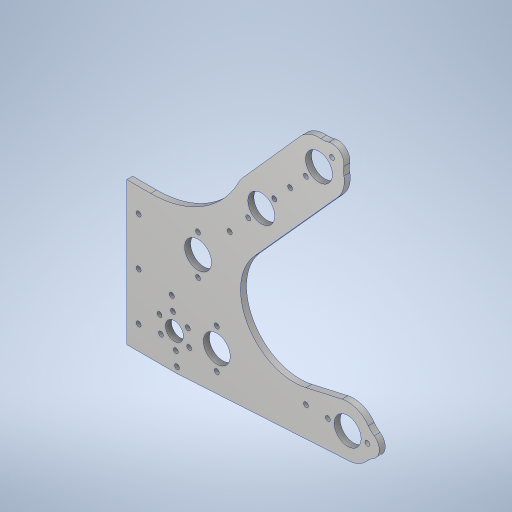
# Autodesk Inventor part: GP8-002
Saved by Autodesk Inventor 2023.4 (Build 274418000, 418)
## iProperties
Created: 2025-02-26
Part Number: GP8-002
Material: Aluminum 6061
Document SubType Name: Modeling
Designer: dlangdon
Density: 2.7 g/cm^3
Appearance: Aluminum - Flat
Author: dlangdon
Autodesk Inventor part; units mm, degrees
ref_plane "YZ Plane" through (0, 0, 0) normal (1, 0, 0) x (0, 1, 0)
ref_plane "XZ Plane" through (0, 0, 0) normal (0, 1, 0) x (-1, 0, 0)
ref_plane "XY Plane" through (0, 0, 0) normal (0, 0, 1) x (1, 0, 0)
sketch "Sketch1" plane through (0, 0, 0) normal (0, 0, 1) x (1, 0, 0)
  line L0 (0, 0) -> (704.681, 0) construction
  line L1 (704.681, 0) -> (704.681, 101.6) construction
  line L2 (704.681, 101.6) -> (0, 101.6) construction
  circle A0 centre (304.8, 38.1) radius 38.1 construction
  circle A1 centre (212.725, 197.5786) radius 38.1 construction
  circle A2 centre (274.2046, 266.7) radius 38.1 construction
  circle A3 centre (499.5893, 180.5177) radius 203.2 construction
  line L3 (78.3329, 304.8) -> (550.894, 304.8) construction
  circle A4 centre (247.764, 111.4893) radius 57.15 construction
  circle A5 centre (258.7625, 117.8393) radius 53.975 construction
  line L4 (212.725, 197.5786) -> (304.8, 38.1) construction
  line L5 (258.7625, 117.8393) -> (247.764, 111.4893) construction
  line L6 (274.2046, 266.7) -> (212.725, 197.5786) construction
  dimension "d0" = 101.6
  dimension "d2" = 76.2
  dimension "d3" = 76.2
  dimension "d4" = 76.2
  dimension "d8" = 406.4
  dimension "d9" = 304.8
  dimension "d11" = 304.8
  dimension "d13" = 114.3
  dimension "d14" = 107.95
  dimension "d15" = 12.7
  dimension "d16" = 92.5068
  dimension "d17" = 60
  constraints: 14 end point, 6 centre point, 6 tangent, 3 perpendicular, 2 horizontal, 1 midpoint
  measures "d0" distance of L0.end L1.end
  measures "d2" diameter of A0
  measures "d3" diameter of A1
  measures "d4" diameter of A2
  measures "d8" diameter of A3
  measures "d9" distance between parallel lines of L0 L3
  measures "d11" horizontal distance of L4.end L0.start
  measures "d13" diameter of A4
  measures "d14" diameter of A5
  measures "d15" distance of L5.start L5.end
  measures "d16" distance of L6.start L4.start
  measures "d17" angle of L0 L4
sketch "Sketch4" plane through (0, 0, 0) normal (0, 0, 1) x (1, 0, 0)
  circle A0 centre (274.2046, 266.7) radius 38.1 construction
  circle A1 centre (212.725, 197.5786) radius 38.1 construction
  circle A2 centre (247.764, 111.4893) radius 57.15 construction
  circle A3 centre (304.8, 38.1) radius 38.1 construction
  circle A4 centre (274.2046, 266.7) radius 14.2875
  circle A5 centre (212.725, 197.5786) radius 14.2875
  circle A6 centre (304.8, 38.1) radius 14.2875
  circle A7 centre (145.2547, 121.0056) radius 39.6875 construction
  circle A8 centre (165.2583, 44.1925) radius 39.6875 construction
  circle A9 centre (145.2547, 121.0056) radius 14.2875
  circle A10 centre (165.2583, 44.1925) radius 14.2875
  line L0 (304.8, 38.1) -> (165.2583, 44.1925) construction
  line L1 (145.2547, 121.0056) -> (212.725, 197.5786) construction
  circle A11 centre (165.2583, 44.1925) radius 23.876 construction
  circle A12 centre (145.2547, 121.0056) radius 23.876 construction
  line L2 (128.9029, 138.4033) -> (202.94, 207.9895) construction
  line L3 (164.5725, 106.974) -> (224.2849, 189.182) construction
  line L4 (165.8568, 20.324) -> (305.1581, 23.817) construction
  line L5 (306.4016, 52.2974) -> (167.9348, 67.918) construction
  circle A13 centre (120.0426, 37.9792) radius 5.9531 construction
  circle A14 centre (120.0426, 37.9792) radius 25.4 construction
  circle A15 centre (117.2754, 69.6084) radius 6.35 construction
  circle A16 centre (122.8098, 6.35) radius 6.35 construction
  line L6 (117.2754, 69.6084) -> (122.8098, 6.35) construction
  line L7 (0, 0) -> (304.8, 0) construction
  line L8 (69.2426, 0) -> (94.6426, 0) construction
  line L9 (94.6426, 0) -> (94.6426, 152.4) construction
  line L10 (94.6426, 152.4) -> (69.2426, 152.4)
  line L11 (69.2426, 152.4) -> (69.2426, 0)
  line L12 (81.9426, 127) -> (81.9426, 25.4) construction
  line L13 (283.8015, 39.0168) -> (325.7985, 37.1832) construction
  line L14 (260.2358, 250.9949) -> (288.1734, 282.4051) construction
  line L15 (145.2547, 99.9871) -> (145.2547, 142.0241) construction
  line L16 (165.2583, 23.174) -> (165.2583, 65.211) construction
  line L17 (226.6204, 213.3487) -> (198.8296, 181.8085) construction
  circle A17 centre (304.8, 38.1) radius 26.9875 construction
  circle A18 centre (325.7985, 37.1832) radius 12.7 construction
  circle A19 centre (288.1734, 282.4051) radius 12.7 construction
  line L18 (274.2046, 266.7) -> (212.725, 197.5786) construction
  circle A20 centre (274.2046, 266.7) radius 26.9875 construction
  circle A21 centre (212.725, 197.5786) radius 26.9875 construction
  arc A22 (94.6426, 152.4) -> (188.7085, 209.8884) centre (94.6426, 258.1022) ccw
  line L19 (254.0394, 284.6358) -> (192.5598, 215.5143)
  arc A23 (280.9291, 292.8363) -> (254.0394, 284.6358) centre (274.2046, 266.7) ccw
  arc A24 (299.3783, 276.4268) -> (280.9291, 292.8363) centre (288.1734, 282.4051) ccw
  line L20 (205.2733, 149.7079) -> (294.2696, 248.6523)
  arc A25 (205.2733, 149.7079) -> (260.3346, 55.7389) centre (247.764, 111.4893) ccw
  line L21 (260.3346, 55.7389) -> (298.8639, 64.4266)
  arc A26 (294.2696, 248.6523) -> (299.3783, 276.4268) centre (274.2046, 266.7) ccw
  arc A27 (192.5598, 215.5143) -> (188.7085, 209.8884) centre (212.725, 197.5786) ccw
  arc A28 (329.3139, 49.387) -> (298.8639, 64.4266) centre (304.8, 38.1) ccw
  arc A29 (328.2369, 24.7195) -> (329.3139, 49.387) centre (325.7985, 37.1832) ccw
  line L22 (306.4392, 11.1623) -> (123.1955, 0.0117)
  line L23 (69.2426, 0) -> (122.8098, 0)
  arc A30 (122.8098, 0) -> (123.1955, 0.0117) centre (122.8098, 6.35) ccw
  arc A31 (306.4392, 11.1623) -> (328.2369, 24.7195) centre (304.8, 38.1) ccw
  circle A32 centre (120.0426, 37.9792) radius 9.525
  circle A33 centre (120.0426, 37.9792) radius 17.4625 construction
  circle A34 centre (260.3923, 40.0389) radius 6.35 construction
  point P0 (81.9426, 76.2)
  point P1 (94.6426, 76.2)
  point P2 (81.9426, 152.4)
  point P3 (243.4648, 232.1393)
  point P4 (118.5207, 55.3752)
  point P5 (178.9898, 159.2921)
  point P6 (104.2162, 45.3592)
  point P7 (105.7382, 27.9631)
  point P8 (121.5646, 20.5831)
  point P9 (135.869, 30.5992)
  point P10 (134.3471, 47.9953)
  dimension "d81" = 34.925
  dimension "d63" = 28.575
  dimension "d64" = 79.375
  dimension "d65" = 47.752
  dimension "d66" = 139.6746
  dimension "d67" = 102.0572
  dimension "d68" = 11.9062
  dimension "d69" = 50.8
  dimension "d70" = 12.7
  dimension "d71" = 2.5
  dimension "d72" = 85
  dimension "d73" = 25.4
  dimension "d74" = 152.4
  dimension "d75" = 101.6
  dimension "d76" = 42.037
  dimension "d77" = 12.7
  dimension "d79" = 25.4
  dimension "d80" = 19.05
  dimension "d92" = 12.7
  dimension "d95" = 360
  constraints: 48 end point, 44 point on circle, 38 coincident, 30 centre point, 22 tangent, 13 equal radius, 11 midpoint, 4 equal length, 4 point on line, 3 collinear, 3 vertical, 2 horizontal, 2 parallel, 2 vertical alignment, 1 concentric, 1 horizontal alignment, 1 perpendicular, 12 other
  measures "d63" diameter of A4
  measures "d64" diameter of A7
  measures "d65" diameter of A11
  measures "d66" distance of L0.end L0.start
  measures "d67" distance of L1.start L1.end
  measures "d68" diameter of A13
  measures "d69" diameter of A14
  measures "d70" diameter of A15
  measures "d71" angle of L7 L0
  measures "d72" angle of L7 L6
  measures "d73" distance of L10.end L9.end
  measures "d74" distance of L9.end L8.end
  measures "d75" distance of L12.start L12.end
  measures "d76" distance of L13.start L13.end
  measures "d77" radial gap between concentric circles of A6 A17
  measures "d79" diameter of A18
  measures "d80" diameter of A32
  measures "d92" diameter of A34
extrude "Extrusion2" add sketch "Sketch4" along normal blind 6.35
hole "Hole2" at (117.2754, 69.6084, 0) at (122.8098, 6.35, 0) at (81.9426, 127, 0) at (81.9426, 76.2, 0) at (81.9426, 25.4, 0) at (283.8015, 39.0168, 0) at (325.7985, 37.1832, 0) at (260.2358, 250.9949, 0) at (288.1734, 282.4051, 0) at (145.2547, 142.0241, 0) at (145.2547, 99.9871, 0) at (165.2583, 65.211, 0) at (165.2583, 23.174, 0) at (198.8296, 181.8085, 0) at (226.6204, 213.3487, 0) at (243.4648, 232.1393, 0) at (118.5207, 55.3752, 0) at (260.3923, 40.0389, 0) at (178.9898, 159.2921, 0) at (134.3471, 47.9953, 0) at (135.869, 30.5992, 0) at (121.5646, 20.5831, 0) at (105.7382, 27.9631, 0) at (104.2162, 45.3592, 0) direction (0, 0, 1) diameter 5.1054 end through all clearance for "Flat Head Machine Screw (82)" size "#10" standard "Ansi Unified Screw Threads"
fillet "Fillet2" radius 25.4 4 edges at (299.3783, 276.4268, 3.175) (280.9291, 292.8363, 3.175) (329.3139, 49.387, 3.175) (328.2369, 24.7195, 3.175)
body "Solid2"
